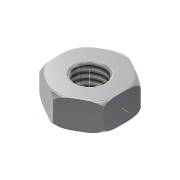
# Autodesk Inventor part: empty
Saved by Autodesk Inventor 2014 (Build 180170000, 170)
## iProperties
Created: 2015-04-13
Part Number: empty
Material: Generic
Document SubType Name: Modeling
Designer: Martin
Density: 1 g/cm^3
Appearance: Default
Author: Martin
Autodesk Inventor part; units mm, degrees
ref_plane "YZ Plane" through (0, 0, 0) normal (1, 0, 0) x (0, 1, 0)
ref_plane "XZ Plane" through (0, 0, 0) normal (0, 1, 0) x (-1, 0, 0)
ref_plane "XY Plane" through (0, 0, 0) normal (0, 0, 1) x (1, 0, 0)
sketch "Sketch1" plane through (0, 0, 0) normal (0, 0, 1) x (1, 0, 0)
  line L0 (0, -4.4456) -> (0, 4.4456) projected
  line L1 (-3.85, 0) -> (3.85, 0) projected
  line L2 (0, 3.1754) -> (-2.75, 1.5877)
  line L3 (-2.75, 1.5877) -> (-2.75, -1.5877)
  line L4 (-2.75, -1.5877) -> (0, -3.1754)
  line L5 (0, -3.1754) -> (2.75, -1.5877)
  line L6 (2.75, -1.5877) -> (2.75, 1.5877)
  line L7 (2.75, 1.5877) -> (0, 3.1754)
  circle A0 centre (0, 0) radius 1.25
  point P0 (-2.75, 0)
  dimension "d2" = 120
  dimension "d3" = 5.5
  dimension "d6" = 2.5
  constraints: 12 end point, 5 equal length, 3 point on line, 1 centre point, 1 coincident, 1 midpoint, 1 parallel, 1 perpendicular
  measures "d2" angle of L7 L2
  measures "d3" distance between parallel lines of L6 L3
  measures "d6" diameter of A0
extrude "Extrusion2" add sketch "Sketch1" along normal mid plane 2.4
extrude "Extrusion3" cut sketch "Sketch1" along normal through all both and the other way through all contours A0 L1 L0 | L0 L1 A0 | L1 A0 L0 | L0 A0 L1
fillet "Fillet1" radius 0.2 2 edges at (-1.25, 0, 1.2) (-1.25, 0, -1.2)
thread "Thread1" size "M3x0.5" class "6H" standard "ANSI Metric M Profile" full length
sketch "Sketch2" plane through (0, 0, 0) normal (1, 0, 0) x (0, 1, 0)
  line L0 (0, -1.6883) -> (0, 1.7297) projected
  line L1 (-3.1754, 1.2) -> (-1.5877, 1.2) projected
  line L2 (-3.1754, -1.2) -> (-3.1754, 1.2) projected
  arc A0 (-2.6754, 1.2) -> (-3.1754, 0.7) centre (-2.6754, 0.7) ccw
  point P0 (0, 0)
  dimension "d14" = 0.5
  constraints: 2 point on circle, 2 point on line, 2 tangent, 1 centre point
  measures "d14" radius of A0
revolve "Revolution1" cut sketch "Sketch2" angle 360 about axis through (0, 0, -10) along (0, 0, 1)
mirror "Mirror1" about plane through (0, 0, 0) normal (0, 0, 1) of "Revolution1"
body "Solid2"
